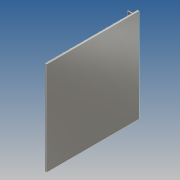
# Autodesk Inventor part: Platina forntal interna
Saved by Autodesk Inventor 2016 (Build 200138000, 138)
## iProperties
Created: 2016-05-25
Part Number: Platina forntal interna
Material: Stainless Steel
Document SubType Name: Modeling
Designer: Familia
Density: 8 g/cm^3
Appearance: Semi-Polished
Mass: 275.6 g
Surface Area: 374.5 cm^2
Volume: 34.45 cm^3
Author: Familia
Autodesk Inventor part; units mm, degrees
ref_plane "YZ Plane" through (0, 0, 0) normal (1, 0, 0) x (0, 1, 0)
ref_plane "XZ Plane" through (0, 0, 0) normal (0, 1, 0) x (-1, 0, 0)
sketch "Sketch1" plane through (0, 0, 0) normal (0, 1, 0) x (-1, 0, 0)
  line L0 (1, 65) -> (-1, 65)
  line L1 (-1, 65) -> (-1, -65)
  line L2 (-1, -65) -> (1, -65)
  line L3 (1, -65) -> (1, 65)
  line L4 (1, 65) -> (-1, -65) construction
  point P0 (0, 0)
  point P1 (0, 0)
  dimension "d0" = 130
  dimension "d1" = 2
  constraints: 10 end point, 2 parallel, 1 coincident, 1 horizontal, 1 midpoint, 1 perpendicular
  measures "d0" distance of L2.end L0.start
  measures "d1" distance of L0.start L0.end
extrude "Extrusion1" add sketch "Sketch1" along normal blind 128
ref_plane "Work Plane1" through (0, 120, 0) normal (0, 1, 0) x (1, 0, 0)
sketch "Sketch2" plane through (0, 120, 0) normal (0, 1, 0) x (1, 0, 0)
  line L0 (-1, -65) -> (1, -65) projected
  line L1 (1, 65) -> (-1, 65) projected
  line L2 (-1, -65) -> (-7, -65)
  line L3 (-7, -65) -> (-7, 65)
  line L4 (-7, 65) -> (-1, 65)
  line L5 (-1, 65) -> (-1, -65)
  point P0 (0, 0)
  dimension "d5" = 6
  constraints: 8 end point, 2 parallel, 1 horizontal, 1 perpendicular
  measures "d5" distance of L0.start L2.end
extrude "Extrusion2" add sketch "Sketch2" along normal blind 1
sketch "Sketch3" plane through (-1, 0, -65) normal (-1, 0, 0) x (0, 0, 1)
  line L0 (0, 5) -> (130, 5)
  line L1 (130, 5) -> (130, 5.5)
  line L2 (130, 5.5) -> (0, 5.5)
  line L3 (0, 5.5) -> (0, 5)
  line L4 (0, 0) -> (0, 120) projected
  line L5 (130, 0) -> (130, 120) projected
  line L6 (0, 0) -> (130, 0) projected
  line L7 (0, 15) -> (130, 15)
  line L8 (130, 15) -> (130, 15.5)
  line L9 (130, 15.5) -> (0, 15.5)
  line L10 (0, 15.5) -> (0, 15)
  line L11 (0, 25) -> (130, 25)
  line L12 (130, 25) -> (130, 25.5)
  line L13 (130, 25.5) -> (0, 25.5)
  line L14 (0, 25.5) -> (0, 25)
  line L15 (0, 35) -> (130, 35)
  line L16 (130, 35) -> (130, 35.5)
  line L17 (130, 35.5) -> (0, 35.5)
  line L18 (0, 35.5) -> (0, 35)
  line L19 (0, 45) -> (130, 45)
  line L20 (130, 45) -> (130, 45.5)
  line L21 (130, 45.5) -> (0, 45.5)
  line L22 (0, 45.5) -> (0, 45)
  line L23 (0, 55) -> (130, 55)
  line L24 (130, 55) -> (130, 55.5)
  line L25 (130, 55.5) -> (0, 55.5)
  line L26 (0, 55.5) -> (0, 55)
  line L27 (0, 65) -> (130, 65)
  line L28 (130, 65) -> (130, 65.5)
  line L29 (130, 65.5) -> (0, 65.5)
  line L30 (0, 65.5) -> (0, 65)
  line L31 (0, 75) -> (130, 75)
  line L32 (130, 75) -> (130, 75.5)
  line L33 (130, 75.5) -> (0, 75.5)
  line L34 (0, 75.5) -> (0, 75)
  line L35 (0, 85) -> (130, 85)
  line L36 (130, 85) -> (130, 85.5)
  line L37 (130, 85.5) -> (0, 85.5)
  line L38 (0, 85.5) -> (0, 85)
  line L39 (0, 95) -> (130, 95)
  line L40 (130, 95) -> (130, 95.5)
  line L41 (130, 95.5) -> (0, 95.5)
  line L42 (0, 95.5) -> (0, 95)
  line L43 (0, 105) -> (130, 105)
  line L44 (130, 105) -> (130, 105.5)
  line L45 (130, 105.5) -> (0, 105.5)
  line L46 (0, 105.5) -> (0, 105)
  line L47 (0, 115) -> (130, 115)
  line L48 (130, 115) -> (130, 115.5)
  line L49 (130, 115.5) -> (0, 115.5)
  line L50 (0, 115.5) -> (0, 115)
  point P0 (65, 0)
  dimension "d8" = 0.5
  dimension "d9" = 5
  dimension "d12" = 10
  constraints: 96 end point, 2 parallel, 2 point on line, 1 horizontal, 1 perpendicular, 1 vertical, 88 other
  measures "d8" distance of L2.end L0.start
  measures "d9" distance between parallel lines of L6 L0
  measures "d12" distance of L0.start L7.start
extrude "Extrusion3" add sketch "Sketch3" along normal blind 0.5 contours L3 L2 L1 L0 | L4 L9 L5 L7 | L4 L13 L5 L11 | L4 L17 L5 L15 | L4 L21 L5 L19 | L4 L25 L5 L23 | L4 L29 L5 L27 | L4 L33 L5 L31 | L4 L37 L5 L35 | L4 L41 L5 L39 | L4 L45 L5 L43 | L4 L49 L5 L47
body "Solid1"
